Autodesk Inventor part; units mm, degrees
(part 2 of 4)
  arc A327 (-798.0511, 322.8727) -> (-803.5503, 322.8727) centre (-800.8007, 321.2852) ccw
  line L333 (-790.8503, 310.4007) -> (-798.0511, 322.8727)
  line L334 (-803.5503, 322.8727) -> (-810.7511, 310.4007)
  arc A328 (-810.7511, 310.4007) -> (-808.0014, 305.6382) centre (-808.0014, 308.8132) ccw
  line L335 (-808.0014, 305.6382) -> (-793.6, 305.6382)
  arc A329 (-793.6, 305.6382) -> (-790.8503, 310.4007) centre (-793.6, 308.8132) ccw
  line L336 (-803.3576, 385.1015) -> (-810.5584, 397.5735)
  arc A330 (-790.6576, 397.5735) -> (-793.4073, 402.336) centre (-793.4073, 399.161) ccw
  arc A331 (-807.8087, 402.336) -> (-810.5584, 397.5735) centre (-807.8087, 399.161) ccw
  arc A332 (-803.3576, 385.1015) -> (-797.8584, 385.1015) centre (-800.608, 386.689) ccw
  line L337 (-790.6576, 397.5735) -> (-797.8584, 385.1015)
  line L338 (-807.8087, 402.336) -> (-793.4073, 402.336)
  arc A333 (-798.0511, 377.2287) -> (-803.5503, 377.2287) centre (-800.8007, 375.6412) ccw
  line L339 (-790.8503, 364.7567) -> (-798.0511, 377.2287)
  line L340 (-803.5503, 377.2287) -> (-810.7511, 364.7567)
  arc A334 (-810.7511, 364.7567) -> (-808.0014, 359.9942) centre (-808.0014, 363.1692) ccw
  line L341 (-808.0014, 359.9942) -> (-793.6, 359.9942)
  arc A335 (-793.6, 359.9942) -> (-790.8503, 364.7567) centre (-793.6, 363.1692) ccw
  line L342 (-749.0016, 58.9655) -> (-756.2024, 71.4375)
  arc A336 (-736.3016, 71.4375) -> (-739.0513, 76.2) centre (-739.0513, 73.025) ccw
  arc A337 (-753.4527, 76.2) -> (-756.2024, 71.4375) centre (-753.4527, 73.025) ccw
  arc A338 (-749.0016, 58.9655) -> (-743.5024, 58.9655) centre (-746.252, 60.553) ccw
  line L343 (-736.3016, 71.4375) -> (-743.5024, 58.9655)
  line L344 (-753.4527, 76.2) -> (-739.0513, 76.2)
  arc A339 (-743.6951, 51.0927) -> (-749.1943, 51.0927) centre (-746.4447, 49.5052) ccw
  line L345 (-736.4943, 38.6207) -> (-743.6951, 51.0927)
  line L346 (-749.1943, 51.0927) -> (-756.3951, 38.6207)
  arc A340 (-756.3951, 38.6207) -> (-753.6454, 33.8582) centre (-753.6454, 37.0332) ccw
  line L347 (-753.6454, 33.8582) -> (-739.244, 33.8582)
  arc A341 (-739.244, 33.8582) -> (-736.4943, 38.6207) centre (-739.244, 37.0332) ccw
  line L348 (-749.0016, 113.3215) -> (-756.2024, 125.7935)
  arc A342 (-736.3016, 125.7935) -> (-739.0513, 130.556) centre (-739.0513, 127.381) ccw
  arc A343 (-753.4527, 130.556) -> (-756.2024, 125.7935) centre (-753.4527, 127.381) ccw
  arc A344 (-749.0016, 113.3215) -> (-743.5024, 113.3215) centre (-746.252, 114.909) ccw
  line L349 (-736.3016, 125.7935) -> (-743.5024, 113.3215)
  line L350 (-753.4527, 130.556) -> (-739.0513, 130.556)
  arc A345 (-743.6951, 105.4487) -> (-749.1943, 105.4487) centre (-746.4447, 103.8612) ccw
  line L351 (-736.4943, 92.9767) -> (-743.6951, 105.4487)
  line L352 (-749.1943, 105.4487) -> (-756.3951, 92.9767)
  arc A346 (-756.3951, 92.9767) -> (-753.6454, 88.2142) centre (-753.6454, 91.3892) ccw
  line L353 (-753.6454, 88.2142) -> (-739.244, 88.2142)
  arc A347 (-739.244, 88.2142) -> (-736.4943, 92.9767) centre (-739.244, 91.3892) ccw
  line L354 (-749.0016, 167.6775) -> (-756.2024, 180.1495)
  arc A348 (-736.3016, 180.1495) -> (-739.0513, 184.912) centre (-739.0513, 181.737) ccw
  arc A349 (-753.4527, 184.912) -> (-756.2024, 180.1495) centre (-753.4527, 181.737) ccw
  arc A350 (-749.0016, 167.6775) -> (-743.5024, 167.6775) centre (-746.252, 169.265) ccw
  line L355 (-736.3016, 180.1495) -> (-743.5024, 167.6775)
  line L356 (-753.4527, 184.912) -> (-739.0513, 184.912)
  arc A351 (-743.6951, 159.8047) -> (-749.1943, 159.8047) centre (-746.4447, 158.2172) ccw
  line L357 (-736.4943, 147.3327) -> (-743.6951, 159.8047)
  line L358 (-749.1943, 159.8047) -> (-756.3951, 147.3327)
  arc A352 (-756.3951, 147.3327) -> (-753.6454, 142.5702) centre (-753.6454, 145.7452) ccw
  line L359 (-753.6454, 142.5702) -> (-739.244, 142.5702)
  arc A353 (-739.244, 142.5702) -> (-736.4943, 147.3327) centre (-739.244, 145.7452) ccw
  line L360 (-749.0016, 222.0335) -> (-756.2024, 234.5055)
  arc A354 (-736.3016, 234.5055) -> (-739.0513, 239.268) centre (-739.0513, 236.093) ccw
  arc A355 (-753.4527, 239.268) -> (-756.2024, 234.5055) centre (-753.4527, 236.093) ccw
  arc A356 (-749.0016, 222.0335) -> (-743.5024, 222.0335) centre (-746.252, 223.621) ccw
  line L361 (-736.3016, 234.5055) -> (-743.5024, 222.0335)
  line L362 (-753.4527, 239.268) -> (-739.0513, 239.268)
  arc A357 (-743.6951, 214.1607) -> (-749.1943, 214.1607) centre (-746.4447, 212.5732) ccw
  line L363 (-736.4943, 201.6887) -> (-743.6951, 214.1607)
  line L364 (-749.1943, 214.1607) -> (-756.3951, 201.6887)
  arc A358 (-756.3951, 201.6887) -> (-753.6454, 196.9262) centre (-753.6454, 200.1012) ccw
  line L365 (-753.6454, 196.9262) -> (-739.244, 196.9262)
  arc A359 (-739.244, 196.9262) -> (-736.4943, 201.6887) centre (-739.244, 200.1012) ccw
  line L366 (-749.0016, 276.3895) -> (-756.2024, 288.8615)
  arc A360 (-736.3016, 288.8615) -> (-739.0513, 293.624) centre (-739.0513, 290.449) ccw
  arc A361 (-753.4527, 293.624) -> (-756.2024, 288.8615) centre (-753.4527, 290.449) ccw
  arc A362 (-749.0016, 276.3895) -> (-743.5024, 276.3895) centre (-746.252, 277.977) ccw
  line L367 (-736.3016, 288.8615) -> (-743.5024, 276.3895)
  line L368 (-753.4527, 293.624) -> (-739.0513, 293.624)
  arc A363 (-743.6951, 268.5167) -> (-749.1943, 268.5167) centre (-746.4447, 266.9292) ccw
  line L369 (-736.4943, 256.0447) -> (-743.6951, 268.5167)
  line L370 (-749.1943, 268.5167) -> (-756.3951, 256.0447)
  arc A364 (-756.3951, 256.0447) -> (-753.6454, 251.2822) centre (-753.6454, 254.4572) ccw
  line L371 (-753.6454, 251.2822) -> (-739.244, 251.2822)
  arc A365 (-739.244, 251.2822) -> (-736.4943, 256.0447) centre (-739.244, 254.4572) ccw
  line L372 (-749.0016, 330.7455) -> (-756.2024, 343.2175)
  arc A366 (-736.3016, 343.2175) -> (-739.0513, 347.98) centre (-739.0513, 344.805) ccw
  arc A367 (-753.4527, 347.98) -> (-756.2024, 343.2175) centre (-753.4527, 344.805) ccw
  arc A368 (-749.0016, 330.7455) -> (-743.5024, 330.7455) centre (-746.252, 332.333) ccw
  line L373 (-736.3016, 343.2175) -> (-743.5024, 330.7455)
  line L374 (-753.4527, 347.98) -> (-739.0513, 347.98)
  arc A369 (-743.6951, 322.8727) -> (-749.1943, 322.8727) centre (-746.4447, 321.2852) ccw
  line L375 (-736.4943, 310.4007) -> (-743.6951, 322.8727)
  line L376 (-749.1943, 322.8727) -> (-756.3951, 310.4007)
  arc A370 (-756.3951, 310.4007) -> (-753.6454, 305.6382) centre (-753.6454, 308.8132) ccw
  line L377 (-753.6454, 305.6382) -> (-739.244, 305.6382)
  arc A371 (-739.244, 305.6382) -> (-736.4943, 310.4007) centre (-739.244, 308.8132) ccw
  line L378 (-749.0016, 385.1015) -> (-756.2024, 397.5735)
  arc A372 (-736.3016, 397.5735) -> (-739.0513, 402.336) centre (-739.0513, 399.161) ccw
  arc A373 (-753.4527, 402.336) -> (-756.2024, 397.5735) centre (-753.4527, 399.161) ccw
  arc A374 (-749.0016, 385.1015) -> (-743.5024, 385.1015) centre (-746.252, 386.689) ccw
  line L379 (-736.3016, 397.5735) -> (-743.5024, 385.1015)
  line L380 (-753.4527, 402.336) -> (-739.0513, 402.336)
  arc A375 (-743.6951, 377.2287) -> (-749.1943, 377.2287) centre (-746.4447, 375.6412) ccw
  line L381 (-736.4943, 364.7567) -> (-743.6951, 377.2287)
  line L382 (-749.1943, 377.2287) -> (-756.3951, 364.7567)
  arc A376 (-756.3951, 364.7567) -> (-753.6454, 359.9942) centre (-753.6454, 363.1692) ccw
  line L383 (-753.6454, 359.9942) -> (-739.244, 359.9942)
  arc A377 (-739.244, 359.9942) -> (-736.4943, 364.7567) centre (-739.244, 363.1692) ccw
  line L384 (-694.6456, 58.9655) -> (-701.8464, 71.4375)
  arc A378 (-681.9456, 71.4375) -> (-684.6953, 76.2) centre (-684.6953, 73.025) ccw
  arc A379 (-699.0967, 76.2) -> (-701.8464, 71.4375) centre (-699.0967, 73.025) ccw
  arc A380 (-694.6456, 58.9655) -> (-689.1464, 58.9655) centre (-691.896, 60.553) ccw
  line L385 (-681.9456, 71.4375) -> (-689.1464, 58.9655)
  line L386 (-699.0967, 76.2) -> (-684.6953, 76.2)
  arc A381 (-689.3391, 51.0927) -> (-694.8383, 51.0927) centre (-692.0887, 49.5052) ccw
  line L387 (-682.1383, 38.6207) -> (-689.3391, 51.0927)
  line L388 (-694.8383, 51.0927) -> (-702.0391, 38.6207)
  arc A382 (-702.0391, 38.6207) -> (-699.2894, 33.8582) centre (-699.2894, 37.0332) ccw
  line L389 (-699.2894, 33.8582) -> (-684.888, 33.8582)
  arc A383 (-684.888, 33.8582) -> (-682.1383, 38.6207) centre (-684.888, 37.0332) ccw
  line L390 (-694.6456, 113.3215) -> (-701.8464, 125.7935)
  arc A384 (-681.9456, 125.7935) -> (-684.6953, 130.556) centre (-684.6953, 127.381) ccw
  arc A385 (-699.0967, 130.556) -> (-701.8464, 125.7935) centre (-699.0967, 127.381) ccw
  arc A386 (-694.6456, 113.3215) -> (-689.1464, 113.3215) centre (-691.896, 114.909) ccw
  line L391 (-681.9456, 125.7935) -> (-689.1464, 113.3215)
  line L392 (-699.0967, 130.556) -> (-684.6953, 130.556)
  arc A387 (-689.3391, 105.4487) -> (-694.8383, 105.4487) centre (-692.0887, 103.8612) ccw
  line L393 (-682.1383, 92.9767) -> (-689.3391, 105.4487)
  line L394 (-694.8383, 105.4487) -> (-702.0391, 92.9767)
  arc A388 (-702.0391, 92.9767) -> (-699.2894, 88.2142) centre (-699.2894, 91.3892) ccw
  line L395 (-699.2894, 88.2142) -> (-684.888, 88.2142)
  arc A389 (-684.888, 88.2142) -> (-682.1383, 92.9767) centre (-684.888, 91.3892) ccw
  line L396 (-694.6456, 167.6775) -> (-701.8464, 180.1495)
  arc A390 (-681.9456, 180.1495) -> (-684.6953, 184.912) centre (-684.6953, 181.737) ccw
  arc A391 (-699.0967, 184.912) -> (-701.8464, 180.1495) centre (-699.0967, 181.737) ccw
  arc A392 (-694.6456, 167.6775) -> (-689.1464, 167.6775) centre (-691.896, 169.265) ccw
  line L397 (-681.9456, 180.1495) -> (-689.1464, 167.6775)
  line L398 (-699.0967, 184.912) -> (-684.6953, 184.912)
  arc A393 (-689.3391, 159.8047) -> (-694.8383, 159.8047) centre (-692.0887, 158.2172) ccw
  line L399 (-682.1383, 147.3327) -> (-689.3391, 159.8047)
  line L400 (-694.8383, 159.8047) -> (-702.0391, 147.3327)
  arc A394 (-702.0391, 147.3327) -> (-699.2894, 142.5702) centre (-699.2894, 145.7452) ccw
  line L401 (-699.2894, 142.5702) -> (-684.888, 142.5702)
  arc A395 (-684.888, 142.5702) -> (-682.1383, 147.3327) centre (-684.888, 145.7452) ccw
  line L402 (-694.6456, 222.0335) -> (-701.8464, 234.5055)
  arc A396 (-681.9456, 234.5055) -> (-684.6953, 239.268) centre (-684.6953, 236.093) ccw
  arc A397 (-699.0967, 239.268) -> (-701.8464, 234.5055) centre (-699.0967, 236.093) ccw
  arc A398 (-694.6456, 222.0335) -> (-689.1464, 222.0335) centre (-691.896, 223.621) ccw
  line L403 (-681.9456, 234.5055) -> (-689.1464, 222.0335)
  line L404 (-699.0967, 239.268) -> (-684.6953, 239.268)
  arc A399 (-689.3391, 214.1607) -> (-694.8383, 214.1607) centre (-692.0887, 212.5732) ccw
  line L405 (-682.1383, 201.6887) -> (-689.3391, 214.1607)
  line L406 (-694.8383, 214.1607) -> (-702.0391, 201.6887)
  arc A400 (-702.0391, 201.6887) -> (-699.2894, 196.9262) centre (-699.2894, 200.1012) ccw
  line L407 (-699.2894, 196.9262) -> (-684.888, 196.9262)
  arc A401 (-684.888, 196.9262) -> (-682.1383, 201.6887) centre (-684.888, 200.1012) ccw
  line L408 (-694.6456, 276.3895) -> (-701.8464, 288.8615)
  arc A402 (-681.9456, 288.8615) -> (-684.6953, 293.624) centre (-684.6953, 290.449) ccw
  arc A403 (-699.0967, 293.624) -> (-701.8464, 288.8615) centre (-699.0967, 290.449) ccw
  arc A404 (-694.6456, 276.3895) -> (-689.1464, 276.3895) centre (-691.896, 277.977) ccw
  line L409 (-681.9456, 288.8615) -> (-689.1464, 276.3895)
  line L410 (-699.0967, 293.624) -> (-684.6953, 293.624)
  arc A405 (-689.3391, 268.5167) -> (-694.8383, 268.5167) centre (-692.0887, 266.9292) ccw
  line L411 (-682.1383, 256.0447) -> (-689.3391, 268.5167)
  line L412 (-694.8383, 268.5167) -> (-702.0391, 256.0447)
  arc A406 (-702.0391, 256.0447) -> (-699.2894, 251.2822) centre (-699.2894, 254.4572) ccw
  line L413 (-699.2894, 251.2822) -> (-684.888, 251.2822)
  arc A407 (-684.888, 251.2822) -> (-682.1383, 256.0447) centre (-684.888, 254.4572) ccw
  line L414 (-694.6456, 330.7455) -> (-701.8464, 343.2175)
  arc A408 (-681.9456, 343.2175) -> (-684.6953, 347.98) centre (-684.6953, 344.805) ccw
  arc A409 (-699.0967, 347.98) -> (-701.8464, 343.2175) centre (-699.0967, 344.805) ccw
  arc A410 (-694.6456, 330.7455) -> (-689.1464, 330.7455) centre (-691.896, 332.333) ccw
  line L415 (-681.9456, 343.2175) -> (-689.1464, 330.7455)
  line L416 (-699.0967, 347.98) -> (-684.6953, 347.98)
  arc A411 (-689.3391, 322.8727) -> (-694.8383, 322.8727) centre (-692.0887, 321.2852) ccw
  line L417 (-682.1383, 310.4007) -> (-689.3391, 322.8727)
  line L418 (-694.8383, 322.8727) -> (-702.0391, 310.4007)
  arc A412 (-702.0391, 310.4007) -> (-699.2894, 305.6382) centre (-699.2894, 308.8132) ccw
  line L419 (-699.2894, 305.6382) -> (-684.888, 305.6382)
  arc A413 (-684.888, 305.6382) -> (-682.1383, 310.4007) centre (-684.888, 308.8132) ccw
  line L420 (-694.6456, 385.1015) -> (-701.8464, 397.5735)
  arc A414 (-681.9456, 397.5735) -> (-684.6953, 402.336) centre (-684.6953, 399.161) ccw
  arc A415 (-699.0967, 402.336) -> (-701.8464, 397.5735) centre (-699.0967, 399.161) ccw
  arc A416 (-694.6456, 385.1015) -> (-689.1464, 385.1015) centre (-691.896, 386.689) ccw
  line L421 (-681.9456, 397.5735) -> (-689.1464, 385.1015)
  line L422 (-699.0967, 402.336) -> (-684.6953, 402.336)
  arc A417 (-689.3391, 377.2287) -> (-694.8383, 377.2287) centre (-692.0887, 375.6412) ccw
  line L423 (-682.1383, 364.7567) -> (-689.3391, 377.2287)
  line L424 (-694.8383, 377.2287) -> (-702.0391, 364.7567)
  arc A418 (-702.0391, 364.7567) -> (-699.2894, 359.9942) centre (-699.2894, 363.1692) ccw
  line L425 (-699.2894, 359.9942) -> (-684.888, 359.9942)
  arc A419 (-684.888, 359.9942) -> (-682.1383, 364.7567) centre (-684.888, 363.1692) ccw
  line L426 (-640.2896, 58.9655) -> (-647.4904, 71.4375)
  arc A420 (-627.5896, 71.4375) -> (-630.3393, 76.2) centre (-630.3393, 73.025) ccw
  arc A421 (-644.7407, 76.2) -> (-647.4904, 71.4375) centre (-644.7407, 73.025) ccw
  arc A422 (-640.2896, 58.9655) -> (-634.7904, 58.9655) centre (-637.54, 60.553) ccw
  line L427 (-627.5896, 71.4375) -> (-634.7904, 58.9655)
  line L428 (-644.7407, 76.2) -> (-630.3393, 76.2)
  arc A423 (-634.9831, 51.0927) -> (-640.4823, 51.0927) centre (-637.7327, 49.5052) ccw
  line L429 (-627.7823, 38.6207) -> (-634.9831, 51.0927)
  line L430 (-640.4823, 51.0927) -> (-647.6831, 38.6207)
  arc A424 (-647.6831, 38.6207) -> (-644.9334, 33.8582) centre (-644.9334, 37.0332) ccw
  line L431 (-644.9334, 33.8582) -> (-630.532, 33.8582)
  arc A425 (-630.532, 33.8582) -> (-627.7823, 38.6207) centre (-630.532, 37.0332) ccw
  line L432 (-640.2896, 113.3215) -> (-647.4904, 125.7935)
  arc A426 (-627.5896, 125.7935) -> (-630.3393, 130.556) centre (-630.3393, 127.381) ccw
  arc A427 (-644.7407, 130.556) -> (-647.4904, 125.7935) centre (-644.7407, 127.381) ccw
  arc A428 (-640.2896, 113.3215) -> (-634.7904, 113.3215) centre (-637.54, 114.909) ccw
  line L433 (-627.5896, 125.7935) -> (-634.7904, 113.3215)
  line L434 (-644.7407, 130.556) -> (-630.3393, 130.556)
  arc A429 (-634.9831, 105.4487) -> (-640.4823, 105.4487) centre (-637.7327, 103.8612) ccw
  line L435 (-627.7823, 92.9767) -> (-634.9831, 105.4487)
  line L436 (-640.4823, 105.4487) -> (-647.6831, 92.9767)
  arc A430 (-647.6831, 92.9767) -> (-644.9334, 88.2142) centre (-644.9334, 91.3892) ccw
  line L437 (-644.9334, 88.2142) -> (-630.532, 88.2142)
  arc A431 (-630.532, 88.2142) -> (-627.7823, 92.9767) centre (-630.532, 91.3892) ccw
  line L438 (-640.2896, 167.6775) -> (-647.4904, 180.1495)
  arc A432 (-627.5896, 180.1495) -> (-630.3393, 184.912) centre (-630.3393, 181.737) ccw
  arc A433 (-644.7407, 184.912) -> (-647.4904, 180.1495) centre (-644.7407, 181.737) ccw
  arc A434 (-640.2896, 167.6775) -> (-634.7904, 167.6775) centre (-637.54, 169.265) ccw
  line L439 (-627.5896, 180.1495) -> (-634.7904, 167.6775)
  line L440 (-644.7407, 184.912) -> (-630.3393, 184.912)
  arc A435 (-634.9831, 159.8047) -> (-640.4823, 159.8047) centre (-637.7327, 158.2172) ccw
  line L441 (-627.7823, 147.3327) -> (-634.9831, 159.8047)
  line L442 (-640.4823, 159.8047) -> (-647.6831, 147.3327)
  arc A436 (-647.6831, 147.3327) -> (-644.9334, 142.5702) centre (-644.9334, 145.7452) ccw
  line L443 (-644.9334, 142.5702) -> (-630.532, 142.5702)
  arc A437 (-630.532, 142.5702) -> (-627.7823, 147.3327) centre (-630.532, 145.7452) ccw
  line L444 (-640.2896, 222.0335) -> (-647.4904, 234.5055)
  arc A438 (-627.5896, 234.5055) -> (-630.3393, 239.268) centre (-630.3393, 236.093) ccw
  arc A439 (-644.7407, 239.268) -> (-647.4904, 234.5055) centre (-644.7407, 236.093) ccw
  arc A440 (-640.2896, 222.0335) -> (-634.7904, 222.0335) centre (-637.54, 223.621) ccw
  line L445 (-627.5896, 234.5055) -> (-634.7904, 222.0335)
  line L446 (-644.7407, 239.268) -> (-630.3393, 239.268)
  arc A441 (-634.9831, 214.1607) -> (-640.4823, 214.1607) centre (-637.7327, 212.5732) ccw
  line L447 (-627.7823, 201.6887) -> (-634.9831, 214.1607)
  line L448 (-640.4823, 214.1607) -> (-647.6831, 201.6887)
  arc A442 (-647.6831, 201.6887) -> (-644.9334, 196.9262) centre (-644.9334, 200.1012) ccw
  line L449 (-644.9334, 196.9262) -> (-630.532, 196.9262)
  arc A443 (-630.532, 196.9262) -> (-627.7823, 201.6887) centre (-630.532, 200.1012) ccw
  line L450 (-640.2896, 276.3895) -> (-647.4904, 288.8615)
  arc A444 (-627.5896, 288.8615) -> (-630.3393, 293.624) centre (-630.3393, 290.449) ccw
  arc A445 (-644.7407, 293.624) -> (-647.4904, 288.8615) centre (-644.7407, 290.449) ccw
  arc A446 (-640.2896, 276.3895) -> (-634.7904, 276.3895) centre (-637.54, 277.977) ccw
  line L451 (-627.5896, 288.8615) -> (-634.7904, 276.3895)
  line L452 (-644.7407, 293.624) -> (-630.3393, 293.624)
  arc A447 (-634.9831, 268.5167) -> (-640.4823, 268.5167) centre (-637.7327, 266.9292) ccw
  line L453 (-627.7823, 256.0447) -> (-634.9831, 268.5167)
  line L454 (-640.4823, 268.5167) -> (-647.6831, 256.0447)
  arc A448 (-647.6831, 256.0447) -> (-644.9334, 251.2822) centre (-644.9334, 254.4572) ccw
  line L455 (-644.9334, 251.2822) -> (-630.532, 251.2822)
  arc A449 (-630.532, 251.2822) -> (-627.7823, 256.0447) centre (-630.532, 254.4572) ccw
  line L456 (-640.2896, 330.7455) -> (-647.4904, 343.2175)
  arc A450 (-627.5896, 343.2175) -> (-630.3393, 347.98) centre (-630.3393, 344.805) ccw
  arc A451 (-644.7407, 347.98) -> (-647.4904, 343.2175) centre (-644.7407, 344.805) ccw
  arc A452 (-640.2896, 330.7455) -> (-634.7904, 330.7455) centre (-637.54, 332.333) ccw
  line L457 (-627.5896, 343.2175) -> (-634.7904, 330.7455)
  line L458 (-644.7407, 347.98) -> (-630.3393, 347.98)
  arc A453 (-634.9831, 322.8727) -> (-640.4823, 322.8727) centre (-637.7327, 321.2852) ccw
  line L459 (-627.7823, 310.4007) -> (-634.9831, 322.8727)
  line L460 (-640.4823, 322.8727) -> (-647.6831, 310.4007)
  arc A454 (-647.6831, 310.4007) -> (-644.9334, 305.6382) centre (-644.9334, 308.8132) ccw
  line L461 (-644.9334, 305.6382) -> (-630.532, 305.6382)
  arc A455 (-630.532, 305.6382) -> (-627.7823, 310.4007) centre (-630.532, 308.8132) ccw
  line L462 (-640.2896, 385.1015) -> (-647.4904, 397.5735)
  arc A456 (-627.5896, 397.5735) -> (-630.3393, 402.336) centre (-630.3393, 399.161) ccw
  arc A457 (-644.7407, 402.336) -> (-647.4904, 397.5735) centre (-644.7407, 399.161) ccw
  arc A458 (-640.2896, 385.1015) -> (-634.7904, 385.1015) centre (-637.54, 386.689) ccw
  line L463 (-627.5896, 397.5735) -> (-634.7904, 385.1015)
  line L464 (-644.7407, 402.336) -> (-630.3393, 402.336)
  arc A459 (-634.9831, 377.2287) -> (-640.4823, 377.2287) centre (-637.7327, 375.6412) ccw
  line L465 (-627.7823, 364.7567) -> (-634.9831, 377.2287)
  line L466 (-640.4823, 377.2287) -> (-647.6831, 364.7567)
  arc A460 (-647.6831, 364.7567) -> (-644.9334, 359.9942) centre (-644.9334, 363.1692) ccw
  line L467 (-644.9334, 359.9942) -> (-630.532, 359.9942)
  arc A461 (-630.532, 359.9942) -> (-627.7823, 364.7567) centre (-630.532, 363.1692) ccw
  line L468 (-585.9336, 58.9655) -> (-593.1344, 71.4375)
  arc A462 (-573.2336, 71.4375) -> (-575.9833, 76.2) centre (-575.9833, 73.025) ccw
  arc A463 (-590.3847, 76.2) -> (-593.1344, 71.4375) centre (-590.3847, 73.025) ccw
  arc A464 (-585.9336, 58.9655) -> (-580.4344, 58.9655) centre (-583.184, 60.553) ccw
  line L469 (-573.2336, 71.4375) -> (-580.4344, 58.9655)
  line L470 (-590.3847, 76.2) -> (-575.9833, 76.2)
  arc A465 (-580.6271, 51.0927) -> (-586.1263, 51.0927) centre (-583.3767, 49.5052) ccw
  line L471 (-573.4263, 38.6207) -> (-580.6271, 51.0927)
  line L472 (-586.1263, 51.0927) -> (-593.3271, 38.6207)
  arc A466 (-593.3271, 38.6207) -> (-590.5774, 33.8582) centre (-590.5774, 37.0332) ccw
  line L473 (-590.5774, 33.8582) -> (-576.176, 33.8582)
  arc A467 (-576.176, 33.8582) -> (-573.4263, 38.6207) centre (-576.176, 37.0332) ccw
  line L474 (-585.9336, 113.3215) -> (-593.1344, 125.7935)
  arc A468 (-573.2336, 125.7935) -> (-575.9833, 130.556) centre (-575.9833, 127.381) ccw
  arc A469 (-590.3847, 130.556) -> (-593.1344, 125.7935) centre (-590.3847, 127.381) ccw
  arc A470 (-585.9336, 113.3215) -> (-580.4344, 113.3215) centre (-583.184, 114.909) ccw
  line L475 (-573.2336, 125.7935) -> (-580.4344, 113.3215)
  line L476 (-590.3847, 130.556) -> (-575.9833, 130.556)
  arc A471 (-580.6271, 105.4487) -> (-586.1263, 105.4487) centre (-583.3767, 103.8612) ccw
  line L477 (-573.4263, 92.9767) -> (-580.6271, 105.4487)
  line L478 (-586.1263, 105.4487) -> (-593.3271, 92.9767)
  arc A472 (-593.3271, 92.9767) -> (-590.5774, 88.2142) centre (-590.5774, 91.3892) ccw
  line L479 (-590.5774, 88.2142) -> (-576.176, 88.2142)
  arc A473 (-576.176, 88.2142) -> (-573.4263, 92.9767) centre (-576.176, 91.3892) ccw
  line L480 (-585.9336, 167.6775) -> (-593.1344, 180.1495)
  arc A474 (-573.2336, 180.1495) -> (-575.9833, 184.912) centre (-575.9833, 181.737) ccw
  arc A475 (-590.3847, 184.912) -> (-593.1344, 180.1495) centre (-590.3847, 181.737) ccw
  arc A476 (-585.9336, 167.6775) -> (-580.4344, 167.6775) centre (-583.184, 169.265) ccw
  line L481 (-573.2336, 180.1495) -> (-580.4344, 167.6775)
  line L482 (-590.3847, 184.912) -> (-575.9833, 184.912)
  arc A477 (-580.6271, 159.8047) -> (-586.1263, 159.8047) centre (-583.3767, 158.2172) ccw
  line L483 (-573.4263, 147.3327) -> (-580.6271, 159.8047)
  line L484 (-586.1263, 159.8047) -> (-593.3271, 147.3327)
  arc A478 (-593.3271, 147.3327) -> (-590.5774, 142.5702) centre (-590.5774, 145.7452) ccw
  line L485 (-590.5774, 142.5702) -> (-576.176, 142.5702)
  arc A479 (-576.176, 142.5702) -> (-573.4263, 147.3327) centre (-576.176, 145.7452) ccw
  line L486 (-585.9336, 222.0335) -> (-593.1344, 234.5055)
  arc A480 (-573.2336, 234.5055) -> (-575.9833, 239.268) centre (-575.9833, 236.093) ccw
  arc A481 (-590.3847, 239.268) -> (-593.1344, 234.5055) centre (-590.3847, 236.093) ccw
  arc A482 (-585.9336, 222.0335) -> (-580.4344, 222.0335) centre (-583.184, 223.621) ccw
  line L487 (-573.2336, 234.5055) -> (-580.4344, 222.0335)
  line L488 (-590.3847, 239.268) -> (-575.9833, 239.268)
  arc A483 (-580.6271, 214.1607) -> (-586.1263, 214.1607) centre (-583.3767, 212.5732) ccw
  line L489 (-573.4263, 201.6887) -> (-580.6271, 214.1607)
  line L490 (-586.1263, 214.1607) -> (-593.3271, 201.6887)
  arc A484 (-593.3271, 201.6887) -> (-590.5774, 196.9262) centre (-590.5774, 200.1012) ccw
  line L491 (-590.5774, 196.9262) -> (-576.176, 196.9262)
  arc A485 (-576.176, 196.9262) -> (-573.4263, 201.6887) centre (-576.176, 200.1012) ccw
  line L492 (-585.9336, 276.3895) -> (-593.1344, 288.8615)
  arc A486 (-573.2336, 288.8615) -> (-575.9833, 293.624) centre (-575.9833, 290.449) ccw
  arc A487 (-590.3847, 293.624) -> (-593.1344, 288.8615) centre (-590.3847, 290.449) ccw
  arc A488 (-585.9336, 276.3895) -> (-580.4344, 276.3895) centre (-583.184, 277.977) ccw
  line L493 (-573.2336, 288.8615) -> (-580.4344, 276.3895)
  line L494 (-590.3847, 293.624) -> (-575.9833, 293.624)
  arc A489 (-580.6271, 268.5167) -> (-586.1263, 268.5167) centre (-583.3767, 266.9292) ccw
  line L495 (-573.4263, 256.0447) -> (-580.6271, 268.5167)
  line L496 (-586.1263, 268.5167) -> (-593.3271, 256.0447)
  arc A490 (-593.3271, 256.0447) -> (-590.5774, 251.2822) centre (-590.5774, 254.4572) ccw
  line L497 (-590.5774, 251.2822) -> (-576.176, 251.2822)
  arc A491 (-576.176, 251.2822) -> (-573.4263, 256.0447) centre (-576.176, 254.4572) ccw
  line L498 (-585.9336, 330.7455) -> (-593.1344, 343.2175)
  arc A492 (-573.2336, 343.2175) -> (-575.9833, 347.98) centre (-575.9833, 344.805) ccw
  arc A493 (-590.3847, 347.98) -> (-593.1344, 343.2175) centre (-590.3847, 344.805) ccw
  arc A494 (-585.9336, 330.7455) -> (-580.4344, 330.7455) centre (-583.184, 332.333) ccw
  line L499 (-573.2336, 343.2175) -> (-580.4344, 330.7455)
  line L500 (-590.3847, 347.98) -> (-575.9833, 347.98)
  arc A495 (-580.6271, 322.8727) -> (-586.1263, 322.8727) centre (-583.3767, 321.2852) ccw
  line L501 (-573.4263, 310.4007) -> (-580.6271, 322.8727)
  line L502 (-586.1263, 322.8727) -> (-593.3271, 310.4007)
  arc A496 (-593.3271, 310.4007) -> (-590.5774, 305.6382) centre (-590.5774, 308.8132) ccw
  line L503 (-590.5774, 305.6382) -> (-576.176, 305.6382)
  arc A497 (-576.176, 305.6382) -> (-573.4263, 310.4007) centre (-576.176, 308.8132) ccw
  line L504 (-585.9336, 385.1015) -> (-593.1344, 397.5735)
  arc A498 (-573.2336, 397.5735) -> (-575.9833, 402.336) centre (-575.9833, 399.161) ccw
  arc A499 (-590.3847, 402.336) -> (-593.1344, 397.5735) centre (-590.3847, 399.161) ccw
  arc A500 (-585.9336, 385.1015) -> (-580.4344, 385.1015) centre (-583.184, 386.689) ccw
  line L505 (-573.2336, 397.5735) -> (-580.4344, 385.1015)
  line L506 (-590.3847, 402.336) -> (-575.9833, 402.336)
  arc A501 (-580.6271, 377.2287) -> (-586.1263, 377.2287) centre (-583.3767, 375.6412) ccw
  line L507 (-573.4263, 364.7567) -> (-580.6271, 377.2287)
  line L508 (-586.1263, 377.2287) -> (-593.3271, 364.7567)
  arc A502 (-593.3271, 364.7567) -> (-590.5774, 359.9942) centre (-590.5774, 363.1692) ccw
  line L509 (-590.5774, 359.9942) -> (-576.176, 359.9942)
  arc A503 (-576.176, 359.9942) -> (-573.4263, 364.7567) centre (-576.176, 363.1692) ccw
  line L510 (-531.5776, 58.9655) -> (-538.7784, 71.4375)
  arc A504 (-518.8776, 71.4375) -> (-521.6273, 76.2) centre (-521.6273, 73.025) ccw
  arc A505 (-536.0287, 76.2) -> (-538.7784, 71.4375) centre (-536.0287, 73.025) ccw
  arc A506 (-531.5776, 58.9655) -> (-526.0784, 58.9655) centre (-528.828, 60.553) ccw
  line L511 (-518.8776, 71.4375) -> (-526.0784, 58.9655)
  line L512 (-536.0287, 76.2) -> (-521.6273, 76.2)
  arc A507 (-526.2711, 51.0927) -> (-531.7703, 51.0927) centre (-529.0207, 49.5052) ccw
  line L513 (-519.0703, 38.6207) -> (-526.2711, 51.0927)
  line L514 (-531.7703, 51.0927) -> (-538.9711, 38.6207)
  arc A508 (-538.9711, 38.6207) -> (-536.2214, 33.8582) centre (-536.2214, 37.0332) ccw
  line L515 (-536.2214, 33.8582) -> (-521.82, 33.8582)
  arc A509 (-521.82, 33.8582) -> (-519.0703, 38.6207) centre (-521.82, 37.0332) ccw
  line L516 (-531.5776, 113.3215) -> (-538.7784, 125.7935)
  arc A510 (-518.8776, 125.7935) -> (-521.6273, 130.556) centre (-521.6273, 127.381) ccw
  arc A511 (-536.0287, 130.556) -> (-538.7784, 125.7935) centre (-536.0287, 127.381) ccw
  arc A512 (-531.5776, 113.3215) -> (-526.0784, 113.3215) centre (-528.828, 114.909) ccw
  line L517 (-518.8776, 125.7935) -> (-526.0784, 113.3215)
  line L518 (-536.0287, 130.556) -> (-521.6273, 130.556)
  arc A513 (-526.2711, 105.4487) -> (-531.7703, 105.4487) centre (-529.0207, 103.8612) ccw
  line L519 (-519.0703, 92.9767) -> (-526.2711, 105.4487)
  line L520 (-531.7703, 105.4487) -> (-538.9711, 92.9767)
  arc A514 (-538.9711, 92.9767) -> (-536.2214, 88.2142) centre (-536.2214, 91.3892) ccw
  line L521 (-536.2214, 88.2142) -> (-521.82, 88.2142)
  arc A515 (-521.82, 88.2142) -> (-519.0703, 92.9767) centre (-521.82, 91.3892) ccw
  line L522 (-531.5776, 167.6775) -> (-538.7784, 180.1495)
  arc A516 (-518.8776, 180.1495) -> (-521.6273, 184.912) centre (-521.6273, 181.737) ccw
  arc A517 (-536.0287, 184.912) -> (-538.7784, 180.1495) centre (-536.0287, 181.737) ccw
  arc A518 (-531.5776, 167.6775) -> (-526.0784, 167.6775) centre (-528.828, 169.265) ccw
  line L523 (-518.8776, 180.1495) -> (-526.0784, 167.6775)
  line L524 (-536.0287, 184.912) -> (-521.6273, 184.912)
  arc A519 (-526.2711, 159.8047) -> (-531.7703, 159.8047) centre (-529.0207, 158.2172) ccw
  line L525 (-519.0703, 147.3327) -> (-526.2711, 159.8047)
  line L526 (-531.7703, 159.8047) -> (-538.9711, 147.3327)
  arc A520 (-538.9711, 147.3327) -> (-536.2214, 142.5702) centre (-536.2214, 145.7452) ccw
  line L527 (-536.2214, 142.5702) -> (-521.82, 142.5702)
  arc A521 (-521.82, 142.5702) -> (-519.0703, 147.3327) centre (-521.82, 145.7452) ccw
  line L528 (-531.5776, 222.0335) -> (-538.7784, 234.5055)
  arc A522 (-518.8776, 234.5055) -> (-521.6273, 239.268) centre (-521.6273, 236.093) ccw
  arc A523 (-536.0287, 239.268) -> (-538.7784, 234.5055) centre (-536.0287, 236.093) ccw
  arc A524 (-531.5776, 222.0335) -> (-526.0784, 222.0335) centre (-528.828, 223.621) ccw
  line L529 (-518.8776, 234.5055) -> (-526.0784, 222.0335)
  line L530 (-536.0287, 239.268) -> (-521.6273, 239.268)
  arc A525 (-526.2711, 214.1607) -> (-531.7703, 214.1607) centre (-529.0207, 212.5732) ccw
  line L531 (-519.0703, 201.6887) -> (-526.2711, 214.1607)
  line L532 (-531.7703, 214.1607) -> (-538.9711, 201.6887)
  arc A526 (-538.9711, 201.6887) -> (-536.2214, 196.9262) centre (-536.2214, 200.1012) ccw
  line L533 (-536.2214, 196.9262) -> (-521.82, 196.9262)
  arc A527 (-521.82, 196.9262) -> (-519.0703, 201.6887) centre (-521.82, 200.1012) ccw
  line L534 (-531.5776, 276.3895) -> (-538.7784, 288.8615)
  arc A528 (-518.8776, 288.8615) -> (-521.6273, 293.624) centre (-521.6273, 290.449) ccw
  arc A529 (-536.0287, 293.624) -> (-538.7784, 288.8615) centre (-536.0287, 290.449) ccw
  arc A530 (-531.5776, 276.3895) -> (-526.0784, 276.3895) centre (-528.828, 277.977) ccw
  line L535 (-518.8776, 288.8615) -> (-526.0784, 276.3895)
  line L536 (-536.0287, 293.624) -> (-521.6273, 293.624)
  arc A531 (-526.2711, 268.5167) -> (-531.7703, 268.5167) centre (-529.0207, 266.9292) ccw
  line L537 (-519.0703, 256.0447) -> (-526.2711, 268.5167)
  line L538 (-531.7703, 268.5167) -> (-538.9711, 256.0447)
  arc A532 (-538.9711, 256.0447) -> (-536.2214, 251.2822) centre (-536.2214, 254.4572) ccw
  line L539 (-536.2214, 251.2822) -> (-521.82, 251.2822)
  arc A533 (-521.82, 251.2822) -> (-519.0703, 256.0447) centre (-521.82, 254.4572) ccw
  line L540 (-531.5776, 330.7455) -> (-538.7784, 343.2175)
  arc A534 (-518.8776, 343.2175) -> (-521.6273, 347.98) centre (-521.6273, 344.805) ccw
  arc A535 (-536.0287, 347.98) -> (-538.7784, 343.2175) centre (-536.0287, 344.805) ccw
  arc A536 (-531.5776, 330.7455) -> (-526.0784, 330.7455) centre (-528.828, 332.333) ccw
  line L541 (-518.8776, 343.2175) -> (-526.0784, 330.7455)
  line L542 (-536.0287, 347.98) -> (-521.6273, 347.98)
  arc A537 (-526.2711, 322.8727) -> (-531.7703, 322.8727) centre (-529.0207, 321.2852) ccw
  line L543 (-519.0703, 310.4007) -> (-526.2711, 322.8727)
  line L544 (-531.7703, 322.8727) -> (-538.9711, 310.4007)
  arc A538 (-538.9711, 310.4007) -> (-536.2214, 305.6382) centre (-536.2214, 308.8132) ccw
  line L545 (-536.2214, 305.6382) -> (-521.82, 305.6382)
  arc A539 (-521.82, 305.6382) -> (-519.0703, 310.4007) centre (-521.82, 308.8132) ccw
  line L546 (-531.5776, 385.1015) -> (-538.7784, 397.5735)
  arc A540 (-518.8776, 397.5735) -> (-521.6273, 402.336) centre (-521.6273, 399.161) ccw
  arc A541 (-536.0287, 402.336) -> (-538.7784, 397.5735) centre (-536.0287, 399.161) ccw
  arc A542 (-531.5776, 385.1015) -> (-526.0784, 385.1015) centre (-528.828, 386.689) ccw
  line L547 (-518.8776, 397.5735) -> (-526.0784, 385.1015)
  line L548 (-536.0287, 402.336) -> (-521.6273, 402.336)
  arc A543 (-526.2711, 377.2287) -> (-531.7703, 377.2287) centre (-529.0207, 375.6412) ccw
  line L549 (-519.0703, 364.7567) -> (-526.2711, 377.2287)
  line L550 (-531.7703, 377.2287) -> (-538.9711, 364.7567)
  arc A544 (-538.9711, 364.7567) -> (-536.2214, 359.9942) centre (-536.2214, 363.1692) ccw
  line L551 (-536.2214, 359.9942) -> (-521.82, 359.9942)
  arc A545 (-521.82, 359.9942) -> (-519.0703, 364.7567) centre (-521.82, 363.1692) ccw
  line L552 (-477.2216, 58.9655) -> (-484.4224, 71.4375)
  arc A546 (-464.5216, 71.4375) -> (-467.2713, 76.2) centre (-467.2713, 73.025) ccw
  arc A547 (-481.6727, 76.2) -> (-484.4224, 71.4375) centre (-481.6727, 73.025) ccw
  arc A548 (-477.2216, 58.9655) -> (-471.7224, 58.9655) centre (-474.472, 60.553) ccw
  line L553 (-464.5216, 71.4375) -> (-471.7224, 58.9655)
  line L554 (-481.6727, 76.2) -> (-467.2713, 76.2)
  arc A549 (-471.9151, 51.0927) -> (-477.4143, 51.0927) centre (-474.6647, 49.5052) ccw
  line L555 (-464.7143, 38.6207) -> (-471.9151, 51.0927)
  line L556 (-477.4143, 51.0927) -> (-484.6151, 38.6207)
  arc A550 (-484.6151, 38.6207) -> (-481.8654, 33.8582) centre (-481.8654, 37.0332) ccw
  line L557 (-481.8654, 33.8582) -> (-467.464, 33.8582)
  arc A551 (-467.464, 33.8582) -> (-464.7143, 38.6207) centre (-467.464, 37.0332) ccw
  line L558 (-477.2216, 113.3215) -> (-484.4224, 125.7935)
  arc A552 (-464.5216, 125.7935) -> (-467.2713, 130.556) centre (-467.2713, 127.381) ccw
  arc A553 (-481.6727, 130.556) -> (-484.4224, 125.7935) centre (-481.6727, 127.381) ccw
  arc A554 (-477.2216, 113.3215) -> (-471.7224, 113.3215) centre (-474.472, 114.909) ccw
  line L559 (-464.5216, 125.7935) -> (-471.7224, 113.3215)
  line L560 (-481.6727, 130.556) -> (-467.2713, 130.556)
  arc A555 (-471.9151, 105.4487) -> (-477.4143, 105.4487) centre (-474.6647, 103.8612) ccw
  line L561 (-464.7143, 92.9767) -> (-471.9151, 105.4487)
  line L562 (-477.4143, 105.4487) -> (-484.6151, 92.9767)
  arc A556 (-484.6151, 92.9767) -> (-481.8654, 88.2142) centre (-481.8654, 91.3892) ccw
  line L563 (-481.8654, 88.2142) -> (-467.464, 88.2142)
  arc A557 (-467.464, 88.2142) -> (-464.7143, 92.9767) centre (-467.464, 91.3892) ccw
  line L564 (-477.2216, 167.6775) -> (-484.4224, 180.1495)
  arc A558 (-464.5216, 180.1495) -> (-467.2713, 184.912) centre (-467.2713, 181.737) ccw
  arc A559 (-481.6727, 184.912) -> (-484.4224, 180.1495) centre (-481.6727, 181.737) ccw
  arc A560 (-477.2216, 167.6775) -> (-471.7224, 167.6775) centre (-474.472, 169.265) ccw
  line L565 (-464.5216, 180.1495) -> (-471.7224, 167.6775)
  line L566 (-481.6727, 184.912) -> (-467.2713, 184.912)
  arc A561 (-471.9151, 159.8047) -> (-477.4143, 159.8047) centre (-474.6647, 158.2172) ccw
  line L567 (-464.7143, 147.3327) -> (-471.9151, 159.8047)
  line L568 (-477.4143, 159.8047) -> (-484.6151, 147.3327)
  arc A562 (-484.6151, 147.3327) -> (-481.8654, 142.5702) centre (-481.8654, 145.7452) ccw
  line L569 (-481.8654, 142.5702) -> (-467.464, 142.5702)
  arc A563 (-467.464, 142.5702) -> (-464.7143, 147.3327) centre (-467.464, 145.7452) ccw
  line L570 (-477.2216, 222.0335) -> (-484.4224, 234.5055)
  arc A564 (-464.5216, 234.5055) -> (-467.2713, 239.268) centre (-467.2713, 236.093) ccw
  arc A565 (-481.6727, 239.268) -> (-484.4224, 234.5055) centre (-481.6727, 236.093) ccw
  arc A566 (-477.2216, 222.0335) -> (-471.7224, 222.0335) centre (-474.472, 223.621) ccw
  line L571 (-464.5216, 234.5055) -> (-471.7224, 222.0335)
  line L572 (-481.6727, 239.268) -> (-467.2713, 239.268)
  arc A567 (-471.9151, 214.1607) -> (-477.4143, 214.1607) centre (-474.6647, 212.5732) ccw
  line L573 (-464.7143, 201.6887) -> (-471.9151, 214.1607)
  line L574 (-477.4143, 214.1607) -> (-484.6151, 201.6887)
  arc A568 (-484.6151, 201.6887) -> (-481.8654, 196.9262) centre (-481.8654, 200.1012) ccw
  line L575 (-481.8654, 196.9262) -> (-467.464, 196.9262)
  arc A569 (-467.464, 196.9262) -> (-464.7143, 201.6887) centre (-467.464, 200.1012) ccw
  line L576 (-477.2216, 276.3895) -> (-484.4224, 288.8615)
  arc A570 (-464.5216, 288.8615) -> (-467.2713, 293.624) centre (-467.2713, 290.449) ccw
  arc A571 (-481.6727, 293.624) -> (-484.4224, 288.8615) centre (-481.6727, 290.449) ccw
  arc A572 (-477.2216, 276.3895) -> (-471.7224, 276.3895) centre (-474.472, 277.977) ccw
  line L577 (-464.5216, 288.8615) -> (-471.7224, 276.3895)
  line L578 (-481.6727, 293.624) -> (-467.2713, 293.624)
  arc A573 (-471.9151, 268.5167) -> (-477.4143, 268.5167) centre (-474.6647, 266.9292) ccw
  line L579 (-464.7143, 256.0447) -> (-471.9151, 268.5167)
  line L580 (-477.4143, 268.5167) -> (-484.6151, 256.0447)
  arc A574 (-484.6151, 256.0447) -> (-481.8654, 251.2822) centre (-481.8654, 254.4572) ccw
  line L581 (-481.8654, 251.2822) -> (-467.464, 251.2822)
  arc A575 (-467.464, 251.2822) -> (-464.7143, 256.0447) centre (-467.464, 254.4572) ccw
  line L582 (-477.2216, 330.7455) -> (-484.4224, 343.2175)
  arc A576 (-464.5216, 343.2175) -> (-467.2713, 347.98) centre (-467.2713, 344.805) ccw
  arc A577 (-481.6727, 347.98) -> (-484.4224, 343.2175) centre (-481.6727, 344.805) ccw
  arc A578 (-477.2216, 330.7455) -> (-471.7224, 330.7455) centre (-474.472, 332.333) ccw
  line L583 (-464.5216, 343.2175) -> (-471.7224, 330.7455)
  line L584 (-481.6727, 347.98) -> (-467.2713, 347.98)
  arc A579 (-471.9151, 322.8727) -> (-477.4143, 322.8727) centre (-474.6647, 321.2852) ccw
  line L585 (-464.7143, 310.4007) -> (-471.9151, 322.8727)
  line L586 (-477.4143, 322.8727) -> (-484.6151, 310.4007)
  arc A580 (-484.6151, 310.4007) -> (-481.8654, 305.6382) centre (-481.8654, 308.8132) ccw
  line L587 (-481.8654, 305.6382) -> (-467.464, 305.6382)
  arc A581 (-467.464, 305.6382) -> (-464.7143, 310.4007) centre (-467.464, 308.8132) ccw
  line L588 (-477.2216, 385.1015) -> (-484.4224, 397.5735)
  arc A582 (-464.5216, 397.5735) -> (-467.2713, 402.336) centre (-467.2713, 399.161) ccw
  arc A583 (-481.6727, 402.336) -> (-484.4224, 397.5735) centre (-481.6727, 399.161) ccw
  arc A584 (-477.2216, 385.1015) -> (-471.7224, 385.1015) centre (-474.472, 386.689) ccw
  line L589 (-464.5216, 397.5735) -> (-471.7224, 385.1015)
  line L590 (-481.6727, 402.336) -> (-467.2713, 402.336)
  arc A585 (-471.9151, 377.2287) -> (-477.4143, 377.2287) centre (-474.6647, 375.6412) ccw
  line L591 (-464.7143, 364.7567) -> (-471.9151, 377.2287)
  line L592 (-477.4143, 377.2287) -> (-484.6151, 364.7567)
  arc A586 (-484.6151, 364.7567) -> (-481.8654, 359.9942) centre (-481.8654, 363.1692) ccw
  line L593 (-481.8654, 359.9942) -> (-467.464, 359.9942)
  arc A587 (-467.464, 359.9942) -> (-464.7143, 364.7567) centre (-467.464, 363.1692) ccw
  line L594 (-422.8656, 58.9655) -> (-430.0664, 71.4375)
  arc A588 (-410.1656, 71.4375) -> (-412.9153, 76.2) centre (-412.9153, 73.025) ccw
  arc A589 (-427.3167, 76.2) -> (-430.0664, 71.4375) centre (-427.3167, 73.025) ccw
  arc A590 (-422.8656, 58.9655) -> (-417.3664, 58.9655) centre (-420.116, 60.553) ccw
  line L595 (-410.1656, 71.4375) -> (-417.3664, 58.9655)
  line L596 (-427.3167, 76.2) -> (-412.9153, 76.2)
  arc A591 (-417.5591, 51.0927) -> (-423.0583, 51.0927) centre (-420.3087, 49.5052) ccw
  line L597 (-410.3583, 38.6207) -> (-417.5591, 51.0927)
  line L598 (-423.0583, 51.0927) -> (-430.2591, 38.6207)
  arc A592 (-430.2591, 38.6207) -> (-427.5094, 33.8582) centre (-427.5094, 37.0332) ccw
  line L599 (-427.5094, 33.8582) -> (-413.108, 33.8582)
  arc A593 (-413.108, 33.8582) -> (-410.3583, 38.6207) centre (-413.108, 37.0332) ccw
  line L600 (-422.8656, 113.3215) -> (-430.0664, 125.7935)
  arc A594 (-410.1656, 125.7935) -> (-412.9153, 130.556) centre (-412.9153, 127.381) ccw
  arc A595 (-427.3167, 130.556) -> (-430.0664, 125.7935) centre (-427.3167, 127.381) ccw
  arc A596 (-422.8656, 113.3215) -> (-417.3664, 113.3215) centre (-420.116, 114.909) ccw
  line L601 (-410.1656, 125.7935) -> (-417.3664, 113.3215)
  line L602 (-427.3167, 130.556) -> (-412.9153, 130.556)
  arc A597 (-417.5591, 105.4487) -> (-423.0583, 105.4487) centre (-420.3087, 103.8612) ccw
  line L603 (-410.3583, 92.9767) -> (-417.5591, 105.4487)
  line L604 (-423.0583, 105.4487) -> (-430.2591, 92.9767)
  arc A598 (-430.2591, 92.9767) -> (-427.5094, 88.2142) centre (-427.5094, 91.3892) ccw
  line L605 (-427.5094, 88.2142) -> (-413.108, 88.2142)
  arc A599 (-413.108, 88.2142) -> (-410.3583, 92.9767) centre (-413.108, 91.3892) ccw
  line L606 (-422.8656, 167.6775) -> (-430.0664, 180.1495)
  arc A600 (-410.1656, 180.1495) -> (-412.9153, 184.912) centre (-412.9153, 181.737) ccw
  arc A601 (-427.3167, 184.912) -> (-430.0664, 180.1495) centre (-427.3167, 181.737) ccw
  arc A602 (-422.8656, 167.6775) -> (-417.3664, 167.6775) centre (-420.116, 169.265) ccw
  line L607 (-410.1656, 180.1495) -> (-417.3664, 167.6775)
  line L608 (-427.3167, 184.912) -> (-412.9153, 184.912)
  arc A603 (-417.5591, 159.8047) -> (-423.0583, 159.8047) centre (-420.3087, 158.2172) ccw
  line L609 (-410.3583, 147.3327) -> (-417.5591, 159.8047)
  line L610 (-423.0583, 159.8047) -> (-430.2591, 147.3327)
  arc A604 (-430.2591, 147.3327) -> (-427.5094, 142.5702) centre (-427.5094, 145.7452) ccw
  line L611 (-427.5094, 142.5702) -> (-413.108, 142.5702)
  arc A605 (-413.108, 142.5702) -> (-410.3583, 147.3327) centre (-413.108, 145.7452) ccw
  line L612 (-422.8656, 222.0335) -> (-430.0664, 234.5055)
  arc A606 (-410.1656, 234.5055) -> (-412.9153, 239.268) centre (-412.9153, 236.093) ccw
  arc A607 (-427.3167, 239.268) -> (-430.0664, 234.5055) centre (-427.3167, 236.093) ccw
  arc A608 (-422.8656, 222.0335) -> (-417.3664, 222.0335) centre (-420.116, 223.621) ccw
  line L613 (-410.1656, 234.5055) -> (-417.3664, 222.0335)
  line L614 (-427.3167, 239.268) -> (-412.9153, 239.268)
  arc A609 (-417.5591, 214.1607) -> (-423.0583, 214.1607) centre (-420.3087, 212.5732) ccw
  line L615 (-410.3583, 201.6887) -> (-417.5591, 214.1607)
  line L616 (-423.0583, 214.1607) -> (-430.2591, 201.6887)
  arc A610 (-430.2591, 201.6887) -> (-427.5094, 196.9262) centre (-427.5094, 200.1012) ccw
  line L617 (-427.5094, 196.9262) -> (-413.108, 196.9262)
  arc A611 (-413.108, 196.9262) -> (-410.3583, 201.6887) centre (-413.108, 200.1012) ccw
  line L618 (-422.8656, 276.3895) -> (-430.0664, 288.8615)
  arc A612 (-410.1656, 288.8615) -> (-412.9153, 293.624) centre (-412.9153, 290.449) ccw
  arc A613 (-427.3167, 293.624) -> (-430.0664, 288.8615) centre (-427.3167, 290.449) ccw
  arc A614 (-422.8656, 276.3895) -> (-417.3664, 276.3895) centre (-420.116, 277.977) ccw
  line L619 (-410.1656, 288.8615) -> (-417.3664, 276.3895)
  line L620 (-427.3167, 293.624) -> (-412.9153, 293.624)
  arc A615 (-417.5591, 268.5167) -> (-423.0583, 268.5167) centre (-420.3087, 266.9292) ccw
  line L621 (-410.3583, 256.0447) -> (-417.5591, 268.5167)
  line L622 (-423.0583, 268.5167) -> (-430.2591, 256.0447)
  arc A616 (-430.2591, 256.0447) -> (-427.5094, 251.2822) centre (-427.5094, 254.4572) ccw
  line L623 (-427.5094, 251.2822) -> (-413.108, 251.2822)
  arc A617 (-413.108, 251.2822) -> (-410.3583, 256.0447) centre (-413.108, 254.4572) ccw
  line L624 (-422.8656, 330.7455) -> (-430.0664, 343.2175)
  arc A618 (-410.1656, 343.2175) -> (-412.9153, 347.98) centre (-412.9153, 344.805) ccw
  arc A619 (-427.3167, 347.98) -> (-430.0664, 343.2175) centre (-427.3167, 344.805) ccw
  arc A620 (-422.8656, 330.7455) -> (-417.3664, 330.7455) centre (-420.116, 332.333) ccw
  line L625 (-410.1656, 343.2175) -> (-417.3664, 330.7455)
  line L626 (-427.3167, 347.98) -> (-412.9153, 347.98)
  arc A621 (-417.5591, 322.8727) -> (-423.0583, 322.8727) centre (-420.3087, 321.2852) ccw
  line L627 (-410.3583, 310.4007) -> (-417.5591, 322.8727)
  line L628 (-423.0583, 322.8727) -> (-430.2591, 310.4007)
  arc A622 (-430.2591, 310.4007) -> (-427.5094, 305.6382) centre (-427.5094, 308.8132) ccw
  line L629 (-427.5094, 305.6382) -> (-413.108, 305.6382)
  arc A623 (-413.108, 305.6382) -> (-410.3583, 310.4007) centre (-413.108, 308.8132) ccw
  line L630 (-422.8656, 385.1015) -> (-430.0664, 397.5735)
  arc A624 (-410.1656, 397.5735) -> (-412.9153, 402.336) centre (-412.9153, 399.161) ccw
  arc A625 (-427.3167, 402.336) -> (-430.0664, 397.5735) centre (-427.3167, 399.161) ccw
  arc A626 (-422.8656, 385.1015) -> (-417.3664, 385.1015) centre (-420.116, 386.689) ccw
  line L631 (-410.1656, 397.5735) -> (-417.3664, 385.1015)
  line L632 (-427.3167, 402.336) -> (-412.9153, 402.336)
  arc A627 (-417.5591, 377.2287) -> (-423.0583, 377.2287) centre (-420.3087, 375.6412) ccw
  line L633 (-410.3583, 364.7567) -> (-417.5591, 377.2287)
  line L634 (-423.0583, 377.2287) -> (-430.2591, 364.7567)
  arc A628 (-430.2591, 364.7567) -> (-427.5094, 359.9942) centre (-427.5094, 363.1692) ccw
  line L635 (-427.5094, 359.9942) -> (-413.108, 359.9942)
  arc A629 (-413.108, 359.9942) -> (-410.3583, 364.7567) centre (-413.108, 363.1692) ccw
  line L636 (-368.5096, 58.9655) -> (-375.7104, 71.4375)
  arc A630 (-355.8096, 71.4375) -> (-358.5593, 76.2) centre (-358.5593, 73.025) ccw
  arc A631 (-372.9607, 76.2) -> (-375.7104, 71.4375) centre (-372.9607, 73.025) ccw
  arc A632 (-368.5096, 58.9655) -> (-363.0104, 58.9655) centre (-365.76, 60.553) ccw
  line L637 (-355.8096, 71.4375) -> (-363.0104, 58.9655)
  line L638 (-372.9607, 76.2) -> (-358.5593, 76.2)
  arc A633 (-363.2031, 51.0927) -> (-368.7023, 51.0927) centre (-365.9527, 49.5052) ccw
  line L639 (-356.0023, 38.6207) -> (-363.2031, 51.0927)
  line L640 (-368.7023, 51.0927) -> (-375.9031, 38.6207)
  arc A634 (-375.9031, 38.6207) -> (-373.1534, 33.8582) centre (-373.1534, 37.0332) ccw
  line L641 (-373.1534, 33.8582) -> (-358.752, 33.8582)
  arc A635 (-358.752, 33.8582) -> (-356.0023, 38.6207) centre (-358.752, 37.0332) ccw
  line L642 (-368.5096, 113.3215) -> (-375.7104, 125.7935)
  arc A636 (-355.8096, 125.7935) -> (-358.5593, 130.556) centre (-358.5593, 127.381) ccw
  arc A637 (-372.9607, 130.556) -> (-375.7104, 125.7935) centre (-372.9607, 127.381) ccw
  arc A638 (-368.5096, 113.3215) -> (-363.0104, 113.3215) centre (-365.76, 114.909) ccw
  line L643 (-355.8096, 125.7935) -> (-363.0104, 113.3215)
  line L644 (-372.9607, 130.556) -> (-358.5593, 130.556)
  arc A639 (-363.2031, 105.4487) -> (-368.7023, 105.4487) centre (-365.9527, 103.8612) ccw
  line L645 (-356.0023, 92.9767) -> (-363.2031, 105.4487)
  line L646 (-368.7023, 105.4487) -> (-375.9031, 92.9767)
  arc A640 (-375.9031, 92.9767) -> (-373.1534, 88.2142) centre (-373.1534, 91.3892) ccw
  line L647 (-373.1534, 88.2142) -> (-358.752, 88.2142)
  arc A641 (-358.752, 88.2142) -> (-356.0023, 92.9767) centre (-358.752, 91.3892) ccw
  line L648 (-368.5096, 167.6775) -> (-375.7104, 180.1495)
  arc A642 (-355.8096, 180.1495) -> (-358.5593, 184.912) centre (-358.5593, 181.737) ccw
  arc A643 (-372.9607, 184.912) -> (-375.7104, 180.1495) centre (-372.9607, 181.737) ccw
  arc A644 (-368.5096, 167.6775) -> (-363.0104, 167.6775) centre (-365.76, 169.265) ccw
  line L649 (-355.8096, 180.1495) -> (-363.0104, 167.6775)
  line L650 (-372.9607, 184.912) -> (-358.5593, 184.912)
  arc A645 (-363.2031, 159.8047) -> (-368.7023, 159.8047) centre (-365.9527, 158.2172) ccw
  line L651 (-356.0023, 147.3327) -> (-363.2031, 159.8047)
  line L652 (-368.7023, 159.8047) -> (-375.9031, 147.3327)
  arc A646 (-375.9031, 147.3327) -> (-373.1534, 142.5702) centre (-373.1534, 145.7452) ccw
  line L653 (-373.1534, 142.5702) -> (-358.752, 142.5702)
  arc A647 (-358.752, 142.5702) -> (-356.0023, 147.3327) centre (-358.752, 145.7452) ccw
  line L654 (-368.5096, 222.0335) -> (-375.7104, 234.5055)
  arc A648 (-355.8096, 234.5055) -> (-358.5593, 239.268) centre (-358.5593, 236.093) ccw
  arc A649 (-372.9607, 239.268) -> (-375.7104, 234.5055) centre (-372.9607, 236.093) ccw
  arc A650 (-368.5096, 222.0335) -> (-363.0104, 222.0335) centre (-365.76, 223.621) ccw
  line L655 (-355.8096, 234.5055) -> (-363.0104, 222.0335)
  line L656 (-372.9607, 239.268) -> (-358.5593, 239.268)
  arc A651 (-363.2031, 214.1607) -> (-368.7023, 214.1607) centre (-365.9527, 212.5732) ccw
  line L657 (-356.0023, 201.6887) -> (-363.2031, 214.1607)
  line L658 (-368.7023, 214.1607) -> (-375.9031, 201.6887)
  arc A652 (-375.9031, 201.6887) -> (-373.1534, 196.9262) centre (-373.1534, 200.1012) ccw
  line L659 (-373.1534, 196.9262) -> (-358.752, 196.9262)
  arc A653 (-358.752, 196.9262) -> (-356.0023, 201.6887) centre (-358.752, 200.1012) ccw
  line L660 (-368.5096, 276.3895) -> (-375.7104, 288.8615)
  arc A654 (-355.8096, 288.8615) -> (-358.5593, 293.624) centre (-358.5593, 290.449) ccw
  arc A655 (-372.9607, 293.624) -> (-375.7104, 288.8615) centre (-372.9607, 290.449) ccw
  arc A656 (-368.5096, 276.3895) -> (-363.0104, 276.3895) centre (-365.76, 277.977) ccw
  line L661 (-355.8096, 288.8615) -> (-363.0104, 276.3895)
  line L662 (-372.9607, 293.624) -> (-358.5593, 293.624)
  arc A657 (-363.2031, 268.5167) -> (-368.7023, 268.5167) centre (-365.9527, 266.9292) ccw
  line L663 (-356.0023, 256.0447) -> (-363.2031, 268.5167)
  line L664 (-368.7023, 268.5167) -> (-375.9031, 256.0447)
  arc A658 (-375.9031, 256.0447) -> (-373.1534, 251.2822) centre (-373.1534, 254.4572) ccw
  line L665 (-373.1534, 251.2822) -> (-358.752, 251.2822)
  arc A659 (-358.752, 251.2822) -> (-356.0023, 256.0447) centre (-358.752, 254.4572) ccw
  line L666 (-368.5096, 330.7455) -> (-375.7104, 343.2175)
  arc A660 (-355.8096, 343.2175) -> (-358.5593, 347.98) centre (-358.5593, 344.805) ccw
  arc A661 (-372.9607, 347.98) -> (-375.7104, 343.2175) centre (-372.9607, 344.805) ccw
  arc A662 (-368.5096, 330.7455) -> (-363.0104, 330.7455) centre (-365.76, 332.333) ccw
  line L667 (-355.8096, 343.2175) -> (-363.0104, 330.7455)
  line L668 (-372.9607, 347.98) -> (-358.5593, 347.98)
  arc A663 (-363.2031, 322.8727) -> (-368.7023, 322.8727) centre (-365.9527, 321.2852) ccw
  line L669 (-356.0023, 310.4007) -> (-363.2031, 322.8727)
  line L670 (-368.7023, 322.8727) -> (-375.9031, 310.4007)
  arc A664 (-375.9031, 310.4007) -> (-373.1534, 305.6382) centre (-373.1534, 308.8132) ccw
  line L671 (-373.1534, 305.6382) -> (-358.752, 305.6382)
  arc A665 (-358.752, 305.6382) -> (-356.0023, 310.4007) centre (-358.752, 308.8132) ccw
  line L672 (-368.5096, 385.1015) -> (-375.7104, 397.5735)
  arc A666 (-355.8096, 397.5735) -> (-358.5593, 402.336) centre (-358.5593, 399.161) ccw